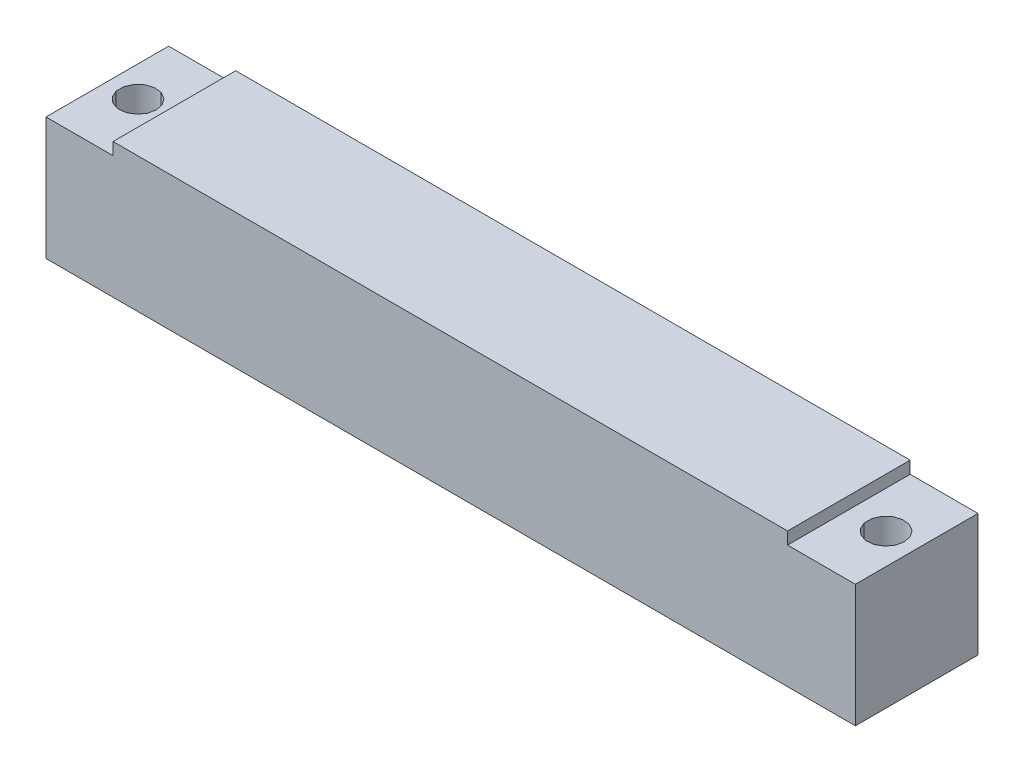
# Autodesk Inventor part: 知能ロボコンラックギア
Saved by Autodesk Inventor 2013 (Build 170138000, 138)
## iProperties
Created: 2014-05-15
Part Number: 知能ロボコンラックギア
Material: 鋼、炭素鋼
Document SubType Name: Modeling
Designer: horumo136
Density: 7.87 g/cm^3
Mass: 56.2015 g
Surface Area: 39.0456 cm^2
Volume: 7.14123 cm^3
Author: horumo136
Autodesk Inventor part; units mm, degrees
ref_plane "YZ Plane" through (0, 0, 0) normal (1, 0, 0) x (0, 1, 0)
ref_plane "XZ Plane" through (0, 0, 0) normal (0, 1, 0) x (-1, 0, 0)
ref_plane "XY Plane" through (0, 0, 0) normal (0, 0, 1) x (1, 0, 0)
sketch "スケッチ1" plane through (0, 0, 0) normal (0, 1, 0) x (-1, 0, 0)
  line L0 (0, 0) -> (-70, 0)
  line L1 (-70, 0) -> (-70, 10)
  line L2 (-70, 10) -> (0, 10)
  line L3 (0, 10) -> (0, 0)
  dimension "d0" = 70
  dimension "d1" = 10
  constraints: 8 end point, 2 parallel, 1 horizontal, 1 perpendicular
  measures "d0" distance of L1.end L2.end
  measures "d1" distance of L0.end L1.end
extrude "押し出し1" add sketch "スケッチ1" along normal blind 10
sketch "スケッチ17" plane through (0, 10, 0) normal (0, 1, 0) x (1, 0, 0)
  line L0 (70, 0) -> (0, 0) projected
  line L1 (0, 0) -> (0, -10) projected
  line L2 (0, -10) -> (70, -10) projected
  line L3 (0, -5) -> (4.5, -5)
  line L4 (4.5, -5) -> (4.5, 0)
  line L5 (70, -5) -> (65.5, -5)
  point P0 (7.0002, -10)
  point P1 (7.0002, 0)
  dimension "d42" = 4.5
  dimension "d43" = 5
  dimension "d44" = 4.5
  dimension "d52" = 61
  constraints: 6 end point, 2 coincident, 2 perpendicular, 1 midpoint, 1 parallel, 1 point on line
  measures "d42" distance of L3.start L3.end
  measures "d43" distance of L3.end L4.end
  measures "d44" distance of L5.start L5.end
  measures "d52" distance of L5.end L3.end
hole "穴1" at (4.5, 10, 5) at (65.5, 10, 5) direction (0, -1, 0) diameter 3 depth 10 tip angle 118
sketch "スケッチ18" plane through (70, 0, 0) normal (0, 0, -1) x (-1, 0, 0)
  line L0 (70, 0) -> (0, 0) projected
  line L1 (0, 10) -> (70, 10) projected
  line L2 (0, 10) -> (2, 10)
  line L3 (2, 10) -> (2, 0)
  line L4 (2, 0) -> (0, 0)
  line L5 (0, 0) -> (0, 10)
  line L6 (70, 0) -> (68, 0)
  line L7 (68, 0) -> (68, 10)
  line L8 (68, 10) -> (70, 10)
  line L9 (70, 10) -> (70, 0)
  point P0 (62.9998, 10)
  dimension "d53" = 2
  dimension "d54" = 2
  constraints: 16 end point, 4 parallel, 2 horizontal, 2 perpendicular, 2 point on line
  measures "d53" distance of L3.end L4.end
  measures "d54" distance of L7.end L8.end
extrude "押し出し15" cut sketch "スケッチ18" against normal blind 10 contours L0 L7 L1 L9 | L0 L5 L1 L3
sketch "スケッチ19" plane through (0, 10, 0) normal (0, 1, 0) x (1, 0, 0)
  line L0 (68, 0) -> (2, 0) projected
  line L1 (2, -10) -> (68, -10) projected
  line L2 (7.4699, 0) -> (62.4699, 0)
  line L3 (62.4699, 0) -> (62.4699, -10)
  line L4 (62.4699, -10) -> (7.4699, -10)
  line L5 (7.4699, -10) -> (7.4699, 0)
  point P0 (0, 0)
  dimension "d57" = 55
  constraints: 8 end point, 2 parallel, 2 point on line, 1 horizontal, 1 perpendicular
  measures "d57" distance of L3.end L4.end
extrude "押し出し16" add sketch "スケッチ19" along normal blind 1
